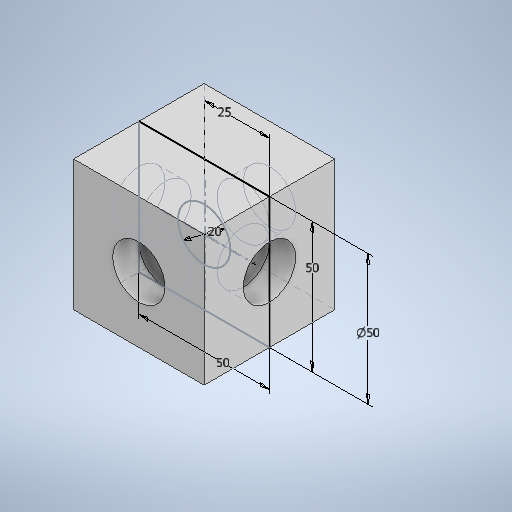
# Autodesk Inventor part: CT_02
Saved by Autodesk Inventor 2025.2 (Build 292293000, 293)
## iProperties
Created: 2024-12-05
Part Number: CT_02
Material: Generic
Document SubType Name: Modeling
Designer: hongquan
Density: 1 g/cm^3
Appearance: Default
Author: hongquan
Autodesk Inventor part; units mm, degrees
ref_plane "YZ Plane" through (0, 0, 0) normal (1, 0, 0) x (0, 1, 0)
ref_plane "XZ Plane" through (0, 0, 0) normal (0, 1, 0) x (-1, 0, 0)
ref_plane "XY Plane" through (0, 0, 0) normal (0, 0, 1) x (1, 0, 0)
sketch "Sketch1" plane through (0, 0, 0) normal (1, 0, 0) x (0, 1, 0)
  line L0 (31.9501, 0) -> (-31.3732, 0)
  line L1 (0, 29.3537) -> (0, -50.8461) construction
  line L2 (25, 25) -> (-25, 25)
  line L3 (-25, 25) -> (-25, -25)
  line L4 (-25, -25) -> (25, -25)
  line L5 (25, -25) -> (25, 25)
  circle A0 centre (0.2885, 0) radius 10
  point P0 (0, 0)
  dimension "d0" = 50
  dimension "d1" = 50
  dimension "d3" = 50
  dimension "d4" = 50
  dimension "d5" = 20
  constraints: 12 end point, 2 horizontal, 2 parallel, 2 vertical, 1 centre point, 1 coincident, 1 midpoint, 1 perpendicular, 1 other
  measures "d0" distance of L2.end L3.end
  measures "d1" distance of L3.end L4.end
  measures "d3" diameter of L4 L0
  measures "d4" diameter of L5 L1
  measures "d5" diameter of A0
sketch "Sketch2" plane through (0, 0, 0) normal (0, 0, 1) x (1, 0, 0)
  line L0 (0, 17.9809) -> (0, -21.5338)
  line L1 (-16.5078, 0) -> (19.6274, 0)
  line L2 (-25, 25) -> (25, 25)
  line L3 (25, 25) -> (25, -25)
  line L4 (25, -25) -> (-25, -25)
  line L5 (-25, -25) -> (-25, 25)
  circle A0 centre (0, 0) radius 10
  dimension "d6" = 50
  dimension "d7" = 50
  dimension "d8" = 25
  dimension "d9" = 50
  dimension "d10" = 20
  constraints: 12 end point, 3 horizontal, 2 parallel, 2 vertical, 1 centre point, 1 coincident, 1 perpendicular
  measures "d6" distance of L3.end L4.end
  measures "d7" distance of L2.end L3.end
  measures "d8" distance from line of L0.start L3
  measures "d9" diameter of L2 L1
  measures "d10" diameter of A0
extrude "Extrusion1" add sketch "Sketch2" along normal mid plane 50
extrude "Extrusion2" add sketch "Sketch2" along normal mid plane 30 contours A0 L1 L0 | L0 L1 A0 | L1 A0 L0 | L0 A0 L1
sketch "Sketch3" plane through (-25, -25, 25) normal (-1, 0, 0) x (0, 0, 1)
  circle A0 centre (-25, 25) radius 10
  dimension "d15" = 20
  constraints: 1 centre point, 1 coincident
  measures "d15" diameter of A0
extrude "Extrusion3" cut sketch "Sketch3" against normal blind 10
sketch "Sketch4" plane through (25, -25, 25) normal (1, 0, 0) x (0, 0, -1)
  circle A0 centre (25, 25) radius 10
  dimension "d18" = 20
  constraints: 1 centre point, 1 coincident
  measures "d18" diameter of A0
extrude "Extrusion4" cut sketch "Sketch4" against normal blind 10
body "Solid1"
